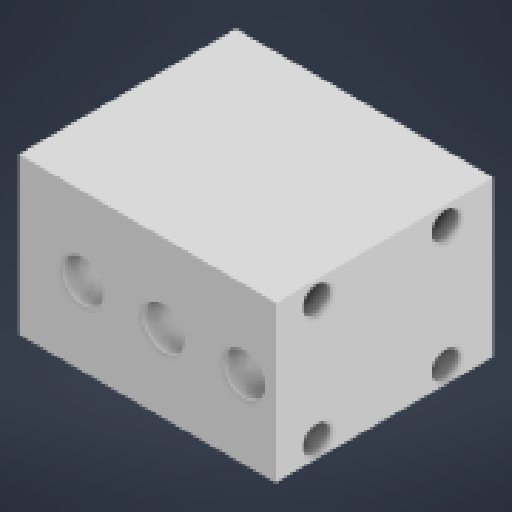
# Autodesk Inventor part: connection block mgn9h
Saved by Autodesk Inventor 2024.3 (Build 283343000, 343)
## iProperties
Created: 2024-11-30
Part Number: connection block mgn9h
Material: Generic
Document SubType Name: Modeling
Designer: MFil
Density: 1 g/cm^3
Appearance: Default
Author: MFil
Autodesk Inventor part; units mm, degrees
ref_plane "YZ Plane" through (0, 0, 0) normal (1, 0, 0) x (0, 1, 0)
ref_plane "XZ Plane" through (0, 0, 0) normal (0, 1, 0) x (-1, 0, 0)
ref_plane "XY Plane" through (0, 0, 0) normal (0, 0, 1) x (1, 0, 0)
sketch "Sketch1" plane through (0, 0, 0) normal (0, 0, 1) x (1, 0, 0)
  circle A0 centre (-50.6259, -62.1376) radius 2.067 projected
  circle A1 centre (-60.6259, -62.1376) radius 2.067 projected
  circle A2 centre (-70.6259, -62.1376) radius 2.067 projected
  arc A3 (-51.6259, -32.7366) -> (-51.6259, -28.7366) centre (-51.6259, -30.7366) ccw projected
  line L0 (-51.6259, -32.7366) -> (-61.6259, -32.7366) projected
  arc A4 (-61.6259, -28.7366) -> (-61.6259, -32.7366) centre (-61.6259, -30.7366) ccw projected
  line L1 (-61.6259, -28.7366) -> (-51.6259, -28.7366) projected
  circle A5 centre (-47.1259, -20.7366) radius 1.2295 projected
  circle A6 centre (-66.1259, -20.7366) radius 1.2295 projected
  circle A7 centre (-47.1259, -10.7366) radius 1.2295 projected
  circle A8 centre (-66.1259, -10.7366) radius 1.2295 projected
  circle A9 centre (-33.2634, 4.8443) radius 1.2295 projected
  circle A10 centre (-15.9429, 14.8443) radius 1.2295 projected
  circle A11 centre (1.3776, 24.8443) radius 1.2295 projected
  circle A12 centre (18.6981, 34.8443) radius 1.2295 projected
  circle A13 centre (36.0187, 44.8443) radius 1.2295 projected
  circle A14 centre (53.3392, 54.8443) radius 1.2295 projected
  circle A15 centre (70.6597, 64.8443) radius 1.2295 projected
  line L2 (72.8006, 71.2078) -> (72.645, 71.1179) projected
  arc A16 (72.645, 71.1179) -> (69.1955, 71.4356) centre (70.6956, 68.8376) ccw projected
  line L3 (69.1955, 71.4356) -> (-42.6259, 6.8679) projected
  line L4 (-42.6259, 6.8679) -> (-42.6259, 0.2634) projected
  arc A17 (-48.6259, -5.7366) -> (-42.6259, 0.2634) centre (-48.6259, 0.2634) ccw projected
  line L5 (-48.6259, -5.7366) -> (-67.6259, -5.7366) projected
  arc A18 (-67.6259, -5.7366) -> (-72.6259, -10.7366) centre (-67.6259, -10.7366) ccw projected
  line L6 (-72.6259, -10.7366) -> (-72.6259, -46.4376) projected
  arc A19 (-78.6259, -52.4376) -> (-72.6259, -46.4376) centre (-78.6259, -46.4376) ccw projected
  line L7 (-78.6259, -52.4376) -> (-78.6259, -71.8376) projected
  line L8 (-78.6259, -71.8376) -> (-48.6259, -71.8376) projected
  arc A20 (-48.6259, -71.8376) -> (-23.6259, -46.8376) centre (-48.6259, -46.8376) ccw projected
  arc A21 (16.3839, 22.4655) -> (-23.6259, -46.8376) centre (56.4008, -46.8376) ccw projected
  line L9 (16.3839, 22.4655) -> (77.126, 57.5391) projected
  arc A22 (77.126, 57.5391) -> (78.2359, 61.6161) centre (75.6259, 60.1371) ccw projected
  line L10 (78.2359, 61.6161) -> (72.8006, 71.2078) projected
  line L11 (-78.6259, -52.4376) -> (-46.6259, -52.4376)
  line L12 (-46.6259, -52.4376) -> (-46.6259, -71.8376)
  line L13 (-46.6259, -71.8376) -> (-78.6259, -71.8376)
  line L14 (-78.6259, -71.8376) -> (-78.6259, -52.4376)
  circle A23 centre (-70.6259, -62.1376) radius 2.6
  circle A24 centre (-60.6259, -62.1376) radius 2.6
  circle A25 centre (-50.6259, -62.1376) radius 2.6
  point P0 (0, 0)
  point P1 (-46.6259, -71.7575)
  dimension "d0" = 32
  dimension "d1" = 19.4
  dimension "d2" = 5.2
  dimension "d3" = 5.2
  dimension "d4" = 5.2
  constraints: 8 end point, 3 centre point, 3 coincident, 2 parallel, 1 horizontal, 1 perpendicular
  measures "d0" distance of L12.end L13.end
  measures "d1" distance of L11.end L12.end
  measures "d2" diameter of A23
  measures "d3" diameter of A24
  measures "d4" diameter of A25
extrude "Extrusion1" add sketch "Sketch1" along normal blind 29 contours L12 L13 A20 | A20 L8 L7 L11 L12
sketch "Sketch2" plane through (-46.6259, -71.7575, 0) normal (1, 0, 0) x (0, 0, -1)
  circle A0 centre (-21.95, 17.1199) radius 1.25
  circle A1 centre (-21.95, 2.1199) radius 1.25
  circle A2 centre (-5.95, 2.1199) radius 1.25
  circle A3 centre (-5.95, 17.1199) radius 1.25
  point P0 (0, 71.7575)
  constraints: 4 centre point
hole "Hole1" at (-46.6259, -69.6376, 21.95) at (-46.6259, -69.6376, 5.95) at (-46.6259, -54.6376, 5.95) at (-46.6259, -54.6376, 21.95) direction (-1, 0, 0) diameter 3.4 end through all clearance for "Countersunk Flat Head Screw ISO 2009/7046" size "M3" standard "ISO"
body "Solid1"
